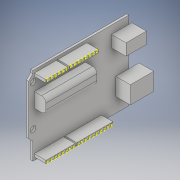
# Autodesk Inventor part: Arduino1
Saved by Autodesk Inventor 2019 (Build 230136000, 136)
## iProperties
Created: 2018-12-19
Part Number: Arduino1
Material: Generic
Document SubType Name: Modeling
Designer: nikol
Density: 1 g/cm^3
Appearance: Default
Author: nikol
Autodesk Inventor part; units mm, degrees
ref_plane "YZ Plane" through (0, 0, 0) normal (1, 0, 0) x (0, 1, 0)
ref_plane "XZ Plane" through (0, 0, 0) normal (0, 1, 0) x (-1, 0, 0)
ref_plane "XY Plane" through (0, 0, 0) normal (0, 0, 1) x (1, 0, 0)
sketch "Sketch1" plane through (0, 0, 0) normal (1, 0, 0) x (0, 1, 0)
  line L0 (27, 34.5) -> (-27, 34.5)
  line L1 (-27, 34.5) -> (-27, -34.5)
  line L2 (-27, -34.5) -> (27, -34.5)
  line L3 (27, -34.5) -> (27, 34.5)
  point P0 (0, 0)
  dimension "d0" = 69
  dimension "d1" = 54
  dimension "d2" = 27
  dimension "d3" = 34.5
  constraints: 8 end point, 2 parallel, 1 horizontal, 1 perpendicular
  measures "d0" distance of L2.end L0.start
  measures "d1" distance of L1.end L2.end
  measures "d2" distance from line of L3 point (0, 0)
  measures "d3" distance from line of L0 point (0, 0)
extrude "Extrusion1" add sketch "Sketch1" along normal blind 1.5
sketch "Sketch3" plane through (1.5, 0, 0) normal (1, 0, 0) x (0, 0, -1)
  line L0 (34.5, 27) -> (-34.5, 27) projected
  line L1 (-31.5, 27) -> (-31.5, 25)
  line L2 (-31.5, 25) -> (-34.5, 22)
  line L3 (-34.5, 22) -> (-37.1788, 22)
  line L4 (-37.1788, 22) -> (-37.1788, 31.2175)
  line L5 (-37.1788, 31.2175) -> (-31.5, 31.2175)
  line L6 (-31.5, 31.2175) -> (-31.5, 27)
  line L7 (-34.5, -27) -> (34.5, -27) projected
  line L8 (-31.5, -27) -> (-31.5, -15)
  line L9 (-31.5, -15) -> (-34.5, -12)
  line L10 (-34.5, -12) -> (-38.8547, -12)
  line L11 (-38.8547, -12) -> (-38.8547, -36.3938)
  line L12 (-38.8547, -36.3938) -> (-31.5, -36.3938)
  line L13 (-31.5, -36.3938) -> (-31.5, -27)
  line L14 (-34.5, 27) -> (-34.5, -27) projected
  point P0 (0, 0)
  dimension "d12" = 3
  dimension "d13" = 12
  dimension "d14" = 3
  dimension "d15" = 3
  dimension "d16" = 2
  constraints: 24 end point, 7 perpendicular, 6 point on line, 2 vertical
  measures "d12" distance between parallel lines of L8 L14
  measures "d13" distance from line of L8.end L7
  measures "d14" horizontal distance of L8.end L9.end
  measures "d15" horizontal distance of L1.end L2.end
  measures "d16" distance from line of L0 L1.end
extrude "Extrusion2" cut sketch "Sketch3" against normal blind 1.5 contours L1 L2 L14 L0 | L9 L8 L7 L14
sketch "Sketch4" plane through (1.5, 0, 0) normal (1, 0, 0) x (0, 0, -1)
  circle A0 centre (-31.5, 20) radius 2
  circle A1 centre (-31.5, -8) radius 2
  line L0 (34.5, 27) -> (-31.5, 27) projected
  line L1 (-34.5, 22) -> (-34.5, -12) projected
  point P0 (0, 0)
  dimension "d19" = 4
  dimension "d20" = 4
  dimension "d21" = 28
  dimension "d22" = 7
  dimension "d25" = 3
  dimension "d26" = 3
  constraints: 2 centre point
  measures "d19" diameter of A0
  measures "d20" diameter of A1
  measures "d21" distance of A0.centre A1.centre
  measures "d22" distance from line of L0 A0.centre
  measures "d25" distance from line of L1 A0.centre
  measures "d26" distance from line of L1 A1.centre
extrude "Extrusion3" cut sketch "Sketch4" against normal blind 1.5
sketch "Sketch5" plane through (1.5, 0, 0) normal (1, 0, 0) x (0, 0, -1)
  line L0 (-30.5, -25) -> (-10.5, -25)
  line L1 (-10.5, -25) -> (-10.5, -23)
  line L2 (-10.5, -23) -> (-30.5, -23)
  line L3 (-30.5, -23) -> (-30.5, -25)
  line L4 (-9.5, -25) -> (15.5, -25)
  line L5 (15.5, -25) -> (15.5, -23)
  line L6 (15.5, -23) -> (-9.5, -23)
  line L7 (-9.5, -23) -> (-9.5, -25)
  line L8 (-30.5, 23) -> (-15.5, 23)
  line L9 (-15.5, 23) -> (-15.5, 25)
  line L10 (-15.5, 25) -> (-30.5, 25)
  line L11 (-30.5, 25) -> (-30.5, 23)
  line L12 (-14.5, 23) -> (5.5, 23)
  line L13 (5.5, 23) -> (5.5, 25)
  line L14 (5.5, 25) -> (-14.5, 25)
  line L15 (-14.5, 25) -> (-14.5, 23)
  line L16 (-31.5, -27) -> (34.5, -27) projected
  line L17 (-31.5, -15) -> (-31.5, -27) projected
  line L18 (34.5, 27) -> (-31.5, 27) projected
  line L19 (-31.5, 27) -> (-31.5, 25) projected
  point P0 (0, 0)
  dimension "d27" = 2
  dimension "d29" = 4
  dimension "d31" = 20
  dimension "d32" = 21
  dimension "d33" = 25
  dimension "d34" = 1
  dimension "d36" = 2
  dimension "d39" = 4
  dimension "d40" = 1
  dimension "d41" = 1
  dimension "d42" = 20
  dimension "d43" = 15
  constraints: 32 end point, 8 parallel, 5 point on line, 4 horizontal, 4 perpendicular
  measures "d27" distance of L0.end L1.end
  measures "d29" distance between parallel lines of L16 L2
  measures "d31" distance of L0.start L0.end
  measures "d32" distance between parallel lines of L17 L1
  measures "d33" distance of L4.start L4.end
  measures "d34" distance between parallel lines of L1 L7
  measures "d36" distance of L10.end L8.start
  measures "d39" distance between parallel lines of L8 L18
  measures "d40" distance between parallel lines of L19 L11
  measures "d41" distance between parallel lines of L9 L15
  measures "d42" distance of L12.start L12.end
  measures "d43" distance of L8.start L8.end
extrude "Extrusion4" add sketch "Sketch5" along normal blind 8
sketch "Sketch6" plane through (9.5, 0, 0) normal (1, 0, 0) x (0, 0, -1)
  line L0 (-30, -24.5) -> (-29, -24.5)
  line L1 (-29, -24.5) -> (-29, -23.5)
  line L2 (-29, -23.5) -> (-30, -23.5)
  line L3 (-30, -23.5) -> (-30, -24.5)
  line L4 (-10.5, -23) -> (-30.5, -23) projected
  line L5 (-30.5, -23) -> (-30.5, -25) projected
  point P0 (0, 0)
  dimension "d46" = 1
  dimension "d47" = 1
  dimension "d48" = 0.5
  dimension "d50" = 1.5
  constraints: 8 end point, 2 parallel, 1 horizontal, 1 perpendicular
  measures "d46" distance between parallel lines of L2 L0
  measures "d47" distance between parallel lines of L1 L3
  measures "d48" distance between parallel lines of L4 L2
  measures "d50" distance between parallel lines of L5 L1
extrude "Extrusion5" cut sketch "Sketch6" against normal blind 5
pattern_linear "Rectangular Pattern1" count 8 spacing 2.54 along (0, 0, -1) of "Extrusion5"
sketch "Sketch7" plane through (9.5, 0, 0) normal (1, 0, 0) x (0, 0, -1)
  line L0 (-9, -24.5) -> (-8, -24.5)
  line L1 (-8, -24.5) -> (-8, -23.5)
  line L2 (-8, -23.5) -> (-9, -23.5)
  line L3 (-9, -23.5) -> (-9, -24.5)
  line L4 (-9.5, -23) -> (-9.5, -25) projected
  line L5 (-9.5, -25) -> (15.5, -25) projected
  point P0 (0, 0)
  dimension "d56" = 0.5
  dimension "d57" = 0.5
  dimension "d58" = 1
  dimension "d59" = 1
  constraints: 8 end point, 2 parallel, 1 horizontal, 1 perpendicular
  measures "d56" distance between parallel lines of L4 L3
  measures "d57" distance between parallel lines of L5 L0
  measures "d58" distance of L0.end L1.end
  measures "d59" distance of L1.end L2.end
extrude "Extrusion6" cut sketch "Sketch7" against normal blind 5
sketch "Sketch8" plane through (9.5, 0, 0) normal (1, 0, 0) x (0, 0, -1)
  line L0 (-13, 24.5) -> (-14, 24.5)
  line L1 (-14, 24.5) -> (-14, 23.5)
  line L2 (-14, 23.5) -> (-13, 23.5)
  line L3 (-13, 23.5) -> (-13, 24.5)
  line L4 (-14.5, 25) -> (-14.5, 23) projected
  line L5 (-14.5, 23) -> (5.5, 23) projected
  point P0 (0, 0)
  dimension "d62" = 0.5
  dimension "d63" = 0.5
  dimension "d64" = 1
  dimension "d65" = 1
  constraints: 8 end point, 2 parallel, 1 horizontal, 1 perpendicular
  measures "d62" distance between parallel lines of L4 L1
  measures "d63" distance between parallel lines of L5 L2
  measures "d64" distance of L1.end L2.end
  measures "d65" distance of L2.end L0.start
extrude "Extrusion7" cut sketch "Sketch8" against normal blind 5
sketch "Sketch9" plane through (9.5, 0, 0) normal (1, 0, 0) x (0, 0, -1)
  line L0 (-29, 24.5) -> (-30, 24.5)
  line L1 (-30, 24.5) -> (-30, 23.5)
  line L2 (-30, 23.5) -> (-29, 23.5)
  line L3 (-29, 23.5) -> (-29, 24.5)
  line L4 (-30.5, 25) -> (-30.5, 23) projected
  line L5 (-30.5, 23) -> (-15.5, 23) projected
  point P0 (0, 0)
  dimension "d68" = 0.5
  dimension "d69" = 0.5
  dimension "d70" = 1
  dimension "d71" = 1
  constraints: 8 end point, 2 parallel, 1 horizontal, 1 perpendicular
  measures "d68" distance between parallel lines of L4 L1
  measures "d69" distance between parallel lines of L5 L2
  measures "d70" distance of L0.start L0.end
  measures "d71" distance of L0.end L1.end
extrude "Extrusion8" cut sketch "Sketch9" against normal blind 5
pattern_linear "Rectangular Pattern2" count 10 spacing 2.54 along (0, 0, -1) of "Extrusion6"
pattern_linear "Rectangular Pattern3" count 6 spacing 2.54 along (0, 0, -1) of "Extrusion8"
pattern_linear "Rectangular Pattern4" count 8 spacing 2.54 along (0, 0, -1) of "Extrusion7"
sketch "Sketch10" plane through (1.5, 0, 0) normal (1, 0, 0) x (0, 0, -1)
  line L0 (-30.5, 14) -> (4.5, 14)
  line L1 (4.5, 14) -> (4.5, 4)
  line L2 (4.5, 4) -> (-30.5, 4)
  line L3 (-30.5, 4) -> (-30.5, 14)
  line L4 (-14.5, 23) -> (5.5, 23) projected
  line L5 (-34.5, 22) -> (-34.5, -12) projected
  point P0 (0, 0)
  dimension "d86" = 9
  dimension "d87" = 10
  dimension "d88" = 35
  dimension "d89" = 4
  constraints: 8 end point, 2 parallel, 1 horizontal, 1 perpendicular
  measures "d86" distance between parallel lines of L4 L0
  measures "d87" distance of L0.end L1.end
  measures "d88" distance of L1.end L2.end
  measures "d89" distance between parallel lines of L5 L3
extrude "Extrusion9" add sketch "Sketch10" along normal blind 8
fillet "Fillet1" radius 3 2 edges at (9.5, 14, 13) (9.5, 4, 13)
sketch "Sketch11" plane through (1.5, 0, 0) normal (1, 0, 0) x (0, 0, -1)
  line L0 (25.5, -17) -> (41.5, -17)
  line L1 (41.5, -17) -> (41.5, -5)
  line L2 (41.5, -5) -> (25.5, -5)
  line L3 (25.5, -5) -> (25.5, -17)
  line L4 (-31.5, -27) -> (34.5, -27) projected
  line L5 (22.5, 21.4458) -> (36.5, 21.4458)
  line L6 (36.5, 21.4458) -> (36.5, 13.4458)
  line L7 (36.5, 13.4458) -> (22.5, 13.4458)
  line L8 (22.5, 13.4458) -> (22.5, 21.4458)
  line L9 (34.5, -27) -> (34.5, 27) projected
  point P0 (0, 0)
  dimension "d93" = 10
  dimension "d94" = 12
  dimension "d95" = 16
  dimension "d96" = 7
  dimension "d97" = 14
  dimension "d98" = 8
  dimension "d99" = 2
  constraints: 16 end point, 4 parallel, 2 horizontal, 2 perpendicular
  measures "d93" distance between parallel lines of L4 L0
  measures "d94" distance of L0.end L1.end
  measures "d95" distance of L1.end L2.end
  measures "d96" distance between parallel lines of L1 L9
  measures "d97" distance of L6.end L7.end
  measures "d98" distance of L5.end L6.end
  measures "d99" distance between parallel lines of L6 L9
extrude "Extrusion10" add sketch "Sketch11" along normal blind 10
sketch "Sketch12" plane through (1.5, 13.4458, -36.5) normal (0, 0, -1) x (-1, 0, 0)
  line L0 (-10, 0) -> (-10, 8) projected
  line L1 (0, 8) -> (-10, 8) projected
  point P0 (1.5, -13.4458)
  point P1 (-6, 4)
  dimension "d109" = 4
  dimension "d110" = 4
  measures "d109" distance from line of L0 point (-6, 4)
  measures "d110" distance from line of L1 point (-6, 4)
hole "Hole1" at (7.5, 17.4458, -36.5) direction (0, 0, 1) diameter 6 depth 8
body "Solid1"
